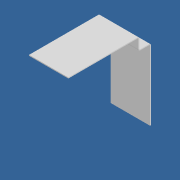
# Autodesk Inventor part: Display_Angle
Saved by Autodesk Inventor 2020 (Build 240168000, 168)
## iProperties
Created: 2021-04-28
Part Number: Display_Angle
Material: 一般
Document SubType Name: Sheet Metal
Designer: ken113
Density: 1 g/cm^3
Sheet Metal Rule: Default_mm
Appearance: 既定
Author: ken113
Autodesk Inventor part; units mm, degrees
ref_plane "YZ Plane" through (0, 0, 0) normal (1, 0, 0) x (0, 1, 0)
ref_plane "XZ Plane" through (0, 0, 0) normal (0, 1, 0) x (-1, 0, 0)
ref_plane "XY Plane" through (0, 0, 0) normal (0, 0, 1) x (1, 0, 0)
sketch "スケッチ1" plane through (0, 0, 0) normal (0, 0, 1) x (1, 0, 0)
  line L0 (-42.5, 0) -> (42.5, 0)
  line L1 (42.5, 0) -> (42.5, -154)
  line L2 (42.5, -154) -> (-42.5, -154)
  line L3 (-42.5, -154) -> (-42.5, 0)
  point P0 (0, 0)
  dimension "d0" = 85
  dimension "d1" = 42.5
  dimension "d2" = 154
  measures "d0" distance of L1.end L2.end
  measures "d1" distance from line of point (0, 0) L3
  measures "d2" distance of L0.end L1.end
extrude "プレート1" add sketch "スケッチ1" along normal blind 2
sketch "スケッチ2" plane through (-42.5, -2, 0) normal (0, 1, 0) x (-1, 0, 0)
  line L0 (-85, 0) -> (0, 0)
  line L1 (0, 0) -> (0, 27)
  line L2 (0, 27) -> (-85, 27)
  line L3 (-85, 27) -> (-85, 0)
  constraints: 6 end point, 1 horizontal, 1 perpendicular, 1 vertical
edge flange "フランジ1" height 27 angle 90 thickness 2 bend radius 2 thickness toward (0, 1, 0) relief straight relief width 2 relief depth 1 edges at (0, 0, 2) wall of the first edge with corners at (42.5, -2, 0) (-42.5, -2, 0) (-42.5, -2, 27) (42.5, -2, 27)
bend "曲げ1"
corner "コーナー1"
sketch "スケッチ3" plane through (42.5, -2, 25) normal (0, 0, 1) x (1, 0, 0)
  line L0 (-85, 0) -> (0, 0)
  line L1 (0, 0) -> (0, 27)
  line L2 (0, 27) -> (-85, 27)
  line L3 (-85, 27) -> (-85, 0)
  constraints: 6 end point, 1 horizontal, 1 perpendicular, 1 vertical
edge flange "フランジ2" height 27 angle 90 thickness 2 bend radius 2 thickness toward (0, 0, 1) relief straight relief width 2 relief depth 1 edges at (0, 0, 27) wall of the first edge with corners at (-42.5, -2, 25) (42.5, -2, 25) (42.5, 25, 25) (-42.5, 25, 25)
bend "曲げ2"
corner "コーナー2"
sketch "スケッチ4" plane through (-42.5, 23, 25) normal (0, 1, 0) x (-1, 0, 0)
  line L0 (-85, 0) -> (0, 0)
  line L1 (0, 0) -> (0, 154)
  line L2 (0, 154) -> (-85, 154)
  line L3 (-85, 154) -> (-85, 0)
  constraints: 6 end point, 1 horizontal, 1 perpendicular, 1 vertical
edge flange "フランジ3" height 154 angle 90 thickness 2 bend radius 2 thickness toward (0, 1, 0) relief straight relief width 2 relief depth 1 edges at (0, 25, 27) wall of the first edge with corners at (42.5, 23, 25) (-42.5, 23, 25) (-42.5, 23, 179) (42.5, 23, 179)
bend "曲げ3"
corner "コーナー3"
equation "\"d3\" = Thickness"
equation "\"d4\" = BendReliefWidth"
equation "\"d5\" = BendReliefDepth"
equation "\"d6\" = MinimumRemnant"
equation "\"d7\" = TransitionRadius"
equation "\"d10\" = BendRadius"
equation "\"d11\" = CornerReliefSize"
equation "\"d12\" = GapSize"
equation "\"d13\" = JacobiRadiusSize"
equation "\"d14\" = BendReliefWidth"
equation "\"d15\" = BendReliefDepth"
equation "\"d16\" = MinimumRemnant"
equation "\"d17\" = TransitionRadius"
equation "\"d20\" = BendRadius"
equation "\"d21\" = CornerReliefSize"
equation "\"d22\" = GapSize"
equation "\"d23\" = JacobiRadiusSize"
equation "\"d24\" = BendReliefWidth"
equation "\"d25\" = BendReliefDepth"
equation "\"d26\" = MinimumRemnant"
equation "\"d27\" = TransitionRadius"
equation "\"d30\" = BendRadius"
equation "\"d31\" = CornerReliefSize"
equation "\"d32\" = GapSize"
equation "\"d33\" = JacobiRadiusSize"
equation "\"BendRadius\" = Thickness"
equation "\"BendReliefWidth\" = Thickness"
equation "\"BendReliefDepth\" = 0.5 * Thickness"
equation "\"CornerReliefSize\" = 4 * Thickness"
equation "\"MinimumRemnant\" = 2 * Thickness"
equation "\"TransitionRadius\" = BendRadius"
equation "\"JacobiRadiusSize\" = BendRadius"
equation "\"GapSize\" = Thickness"
equation "\"Thickness\" = 2"
